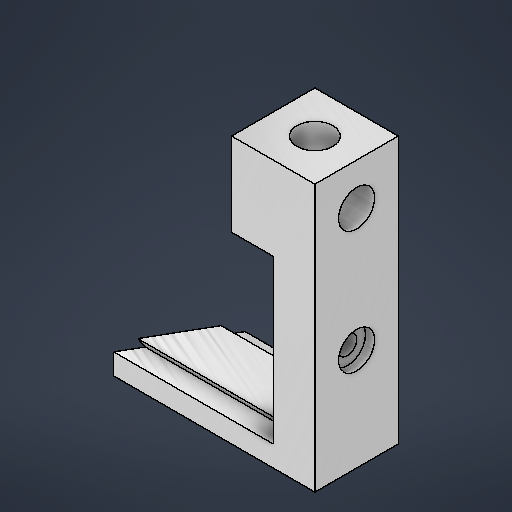
# Autodesk Inventor part: A Idler
Saved by Autodesk Inventor 2026 (Build 300175050, 175E)
## iProperties
Created: 2025-04-15
Part Number: A Idler
Material: Aluminum 6061
Document SubType Name: Modeling
Designer: Joshua Eah
Density: 2.7 g/cm^3
Appearance: Aluminum - Flat
Author: Joshua Eah
Autodesk Inventor part; units mm, degrees
ref_plane "YZ Plane" through (0, 0, 0) normal (1, 0, 0) x (0, 1, 0)
ref_plane "XZ Plane" through (0, 0, 0) normal (0, 1, 0) x (-1, 0, 0)
ref_plane "XY Plane" through (0, 0, 0) normal (0, 0, 1) x (1, 0, 0)
sketch "Overall Profile" plane through (0, 0, 0) normal (0, 1, 0) x (-1, 0, 0)
  line L0 (0, 0) -> (36.2103, 0)
  line L1 (36.2103, 0) -> (36.2103, -15)
  line L2 (36.2103, -15) -> (0, -15)
  line L3 (0, -15) -> (0, 0)
  line L4 (27.55, 0) -> (27.55, -15)
  dimension "d0" = 36.2103
  dimension "d1" = 15
  dimension "d117" = 27.55
  constraints: 10 end point, 2 parallel, 2 perpendicular, 2 point on line, 1 horizontal
  measures "d0" distance of L1.end L2.end
  measures "d1" distance of L0.end L1.end
  measures "d117" distance between parallel lines of L4 L3
extrude "Stock" add sketch "Overall Profile" along normal blind 48
sketch "Top Hole Locations" plane through (0, 48, 0) normal (0, 1, 0) x (1, 0, 0)
  line L0 (0, 15) -> (-36.2103, 15) projected
  line L1 (-36.2103, 15) -> (-36.2103, 0) projected
  line L2 (-36.2103, 0) -> (0, 0) projected
  line L3 (0, 0) -> (0, 15) projected
  line L4 (-36.2103, 0) -> (0, 0) projected
  line L5 (0, 0) -> (-15, 0)
  line L6 (-15, 0) -> (-15, 15)
  line L7 (-15, 15) -> (0, 15)
  line L8 (0, 15) -> (0, 0)
  circle A0 centre (-7.5, 7.5) radius 1.5
  dimension "d72" = 15
  dimension "d83" = 3
  dimension "d84" = 7.5
  dimension "d85" = 7.5
  constraints: 8 end point, 2 parallel, 1 centre point, 1 horizontal, 1 perpendicular, 1 point on line
  measures "d72" distance of L6.end L7.end
  measures "d83" diameter of A0
  measures "d84" distance from line of L3 A0.centre
  measures "d85" distance from line of L0 A0.centre
extrude "Extrusion5" cut sketch "Top Hole Locations" against normal blind 15 contours L6 L2 L1 L0
sketch "Dovetail Slot" plane through (-36.2103, 0, -15) normal (-1, 0, 0) x (0, 0, 1)
  line L0 (15, 0) -> (15, 48) construction
  line L1 (0, 0) -> (0, 33) construction
  line L2 (15, 3.75) -> (0, 3.75)
  line L3 (0, 3.75) -> (0, 33)
  line L4 (0, 33) -> (15, 33)
  line L5 (15, 33) -> (15, 3.75)
  line L6 (0, 0) -> (15, 0) projected
  line L7 (7.5, 33) -> (7.5, 3.75) construction
  line L8 (5.9125, 33) -> (9.0875, 33)
  line L9 (9.0875, 33) -> (9.0875, 31.5)
  line L10 (9.0875, 31.5) -> (5.9125, 31.5)
  line L11 (5.9125, 31.5) -> (5.9125, 33)
  line L12 (2.7375, 3.75) -> (12.2625, 3.75)
  line L13 (12.2625, 3.75) -> (12.2625, 5.25)
  line L14 (12.2625, 5.25) -> (2.7375, 5.25)
  line L15 (2.7375, 5.25) -> (2.7375, 3.75)
  line L16 (2.7375, 5.25) -> (3.6035, 3.75)
  line L17 (2.7375, 5.25) -> (4.4696, 5.25) construction
  line L18 (12.2625, 5.25) -> (11.3965, 3.75)
  line L19 (12.2625, 5.25) -> (13.9946, 5.25) construction
  dimension "d74" = 3.75
  dimension "d75" = 3.175
  dimension "d76" = 1.5875
  dimension "d77" = 1.5
  dimension "d78" = 9.525
  dimension "d79" = 4.7625
  dimension "d80" = 1.5
  dimension "d113" = 60
  dimension "d114" = 120
  constraints: 34 end point, 7 point on line, 6 parallel, 5 horizontal, 3 perpendicular, 2 equal length, 2 midpoint
  measures "d74" distance between parallel lines of L2 L6
  measures "d75" distance between parallel lines of L9 L11
  measures "d76" distance between parallel lines of L9 L7
  measures "d77" distance of L8.end L9.end
  measures "d78" distance between parallel lines of L13 L15
  measures "d79" distance between parallel lines of L7 L15
  measures "d80" distance of L12.end L13.end
  measures "d113" angle of L16 L17
  measures "d114" angle of L18 L19
extrude "Dovetail" cut sketch "Dovetail Slot" against normal blind 28.7103 contours L2 L13 L14 L15 L3 L4 L11 L10 L9 L5 | L2 L18 L13 | L9 L10 L11 L4 | L2 L15 L16
hole "Top Hole" at (-7.5, 48, -7.5) direction (0, -1, 0) diameter 3.4036 end through all counterbore diameter 6.5024 counterbore depth 43 clearance for "Socket Head Cap Screw" size "M3" standard "Ansi Metric M Profile"
sketch "Front Hole Locations" plane through (0, 0, 0) normal (1, 0, 0) x (0, 0, -1)
  circle A0 centre (7.5, 40.5) radius 1.5
  line L0 (0, 48) -> (15, 48) projected
  line L1 (0, 0) -> (0, 48) projected
  circle A1 centre (7.5, 18.375) radius 1.5
  line L2 (0, 3.75) -> (3.6035, 3.75) projected
  line L3 (0, 3.75) -> (3.6035, 3.75) projected
  line L4 (10.7512, 33) -> (4.2488, 33) projected
  line L5 (4.2488, 33) -> (0, 33) projected
  line L6 (15, 33) -> (0, 33) projected
  line L7 (15, 33) -> (10.7512, 33) projected
  point P0 (4.2488, 33)
  dimension "d93" = 3
  dimension "d94" = 7.5
  dimension "d95" = 7.5
  dimension "d103" = 3
  dimension "d104" = 7.5
  dimension "d115" = 29.25
  dimension "d116" = 14.625
  constraints: 2 centre point
  measures "d93" diameter of A0
  measures "d94" distance from line of L0 A0.centre
  measures "d95" distance from line of A0.centre L1
  measures "d103" diameter of A1
  measures "d104" distance from line of L1 A1.centre
  measures "d115" distance between parallel lines of L6 L2
  measures "d116" distance from line of A1.centre L2
hole "Extrusion Mounting Hole" at (0, 40.5, -7.5) direction (-1, 0, 0) diameter 3.4036 end through all counterbore diameter 6.5024 counterbore depth 12 clearance for "Socket Head Cap Screw" size "M3" standard "Ansi Metric M Profile"
hole "Tensioner" at (0, 18.375, -7.5) direction (-1, 0, 0) diameter 3.4036 end through all counterbore diameter 6.5024 counterbore depth 1.65 clearance for "Socket Head Cap Screw" size "M3" standard "Ansi Metric M Profile"
chamfer "Chamfer3" distance 15 angle 30 1 edges at (-36.2103, 1.875, -15) measured on face at (-36.2103, 1.875, -14.5)
equation "\"d84\" = 0.5 * d72"
equation "\"d85\" = 0.5 * d72"
equation "\"d76\" = 0.5 * d75"
equation "\"d79\" = 0.5 * d78"
equation "\"d104\" = d95"
equation "\"d116\" = 0.5 * d115"
body "Solid1"
